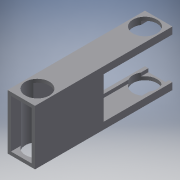
# Autodesk Inventor part: C Arm
Saved by Autodesk Inventor 2018 (Build 220112000, 112)
## iProperties
Created: 2018-01-13
Part Number: C Arm
Material: Generic
Document SubType Name: Modeling
Designer: Orangeracer
Density: 1 g/cm^3
Appearance: Default
Author: Orangeracer
Autodesk Inventor part; units mm, degrees
ref_plane "YZ Plane" through (0, 0, 0) normal (1, 0, 0) x (0, 1, 0)
ref_plane "XZ Plane" through (0, 0, 0) normal (0, 1, 0) x (-1, 0, 0)
ref_plane "XY Plane" through (0, 0, 0) normal (0, 0, 1) x (1, 0, 0)
sketch "Sketch1" plane through (0, 0, 0) normal (0, 0, 1) x (1, 0, 0)
  line L0 (0, 0) -> (25.4, 0)
  line L1 (25.4, 0) -> (25.4, -50.8)
  line L2 (25.4, -50.8) -> (0, -50.8)
  line L3 (0, -50.8) -> (0, 0)
  line L4 (22.225, -3.175) -> (3.175, -3.175)
  line L5 (3.175, -3.175) -> (3.175, -47.625)
  line L6 (3.175, -47.625) -> (22.225, -47.625)
  line L7 (22.225, -47.625) -> (22.225, -3.175)
  dimension "d0" = 25.4
  dimension "d1" = 50.8
  dimension "d2" = 3.175
  constraints: 16 end point, 4 parallel, 2 perpendicular, 1 horizontal, 3 other
  measures "d0" distance of L1.end L2.end
  measures "d1" distance of L0.end L1.end
  measures "d2" distance between parallel lines of L0 L4
extrude "Extrusion1" add sketch "Sketch1" along normal blind 127
sketch "Sketch2" plane through (0, 0, 0) normal (0, 1, 0) x (1, 0, 0)
  circle A0 centre (12.7, -12.7) radius 11.1125
  line L0 (0, 0) -> (0, -127) projected
  line L1 (0, 0) -> (25.4, 0) projected
  circle A1 centre (12.7, -112.0904) radius 11.1125
  circle A2 centre (12.7, -211.4809) radius 11.1125
  dimension "d5" = 12.7
  dimension "d6" = 12.7
  dimension "d7" = 22.225
  dimension "d8" = 99.3904
  dimension "d9" = 99.3904
  dimension "d10" = 12.7
  dimension "d11" = 22.225
  dimension "d12" = 12.7
  dimension "d13" = 22.225
  constraints: 3 centre point
  measures "d5" distance from line of L0 A0.centre
  measures "d6" distance from line of L1 A0.centre
  measures "d7" diameter of A0
  measures "d8" distance of A0.centre A1.centre
  measures "d9" distance of A2.centre A1.centre
  measures "d10" distance from line of L0 A1.centre
  measures "d11" diameter of A1
  measures "d12" distance from line of L0 A2.centre
  measures "d13" diameter of A2
extrude "Extrusion2" cut sketch "Sketch2" against normal blind 127
sketch "Sketch3" plane through (25.4, -50.8, 0) normal (1, 0, 0) x (0, 0, -1)
  line L0 (0, 44.45) -> (-63.5, 44.45)
  line L1 (-63.5, 44.45) -> (-63.5, 6.35)
  line L2 (-63.5, 6.35) -> (0, 6.35)
  line L3 (0, 6.35) -> (0, 44.45)
  line L4 (0, 50.8) -> (-127, 50.8) projected
  line L5 (0, 0) -> (-127, 0) projected
  line L6 (0, 50.8) -> (0, 0) projected
  dimension "d19" = 6.35
  dimension "d20" = 6.35
  dimension "d21" = 38.1
  dimension "d22" = 63.5
  dimension "d23" = 0
  constraints: 8 end point, 2 parallel, 1 horizontal, 1 perpendicular
  measures "d19" distance between parallel lines of L4 L0
  measures "d20" distance between parallel lines of L5 L2
  measures "d21" distance of L0.end L1.end
  measures "d22" distance between parallel lines of L1 L3
  measures "d23" distance between parallel lines of L6 L3
extrude "Extrusion3" cut sketch "Sketch3" against normal blind 127
body "Solid1"
